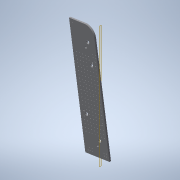
# Autodesk Inventor part: inside wall
Saved by Autodesk Inventor 2020 (Build 240168000, 168)
## iProperties
Created: 2019-10-13
Part Number: inside wall
Material: Generic
Document SubType Name: Modeling
Designer: ball
Density: 1 g/cm^3
Appearance: Default
Author: ball
Autodesk Inventor part; units mm, degrees
ref_plane "XZ Plane" through (0, 0, 0) normal (0, 1, 0) x (-1, 0, 0)
ref_plane "XY Plane" through (0, 0, 0) normal (0, 0, 1) x (1, 0, 0)
ref_plane "Work Plane1" through (-0.0003, 0.0023, 0) normal (0, 0, 1) x (1, 0, 0)
sketch "Sketch1" plane through (-0.0003, 0.0023, 0) normal (0, 0, 1) x (1, 0, 0)
  circle A0 centre (0.0003, -0.0023) radius 6.3373 construction
  circle A1 centre (-49.0975, 326.5271) radius 6.3373 construction
  circle A2 centre (0.0003, -0.0023) radius 6.4516
  circle A3 centre (-49.0975, 326.5271) radius 6.4516
  circle A4 centre (-49.0975, 326.5271) radius 60.325 construction
  circle A5 centre (0.0003, -0.0023) radius 60.325 construction
  circle A6 centre (0.0003, -0.0023) radius 31.75 construction
  circle A7 centre (-49.0975, 326.5271) radius 31.75 construction
  line L0 (-58.7973, -69.8464) -> (40.3672, -54.9357)
  line L1 (-125.8347, 375.9918) -> (-58.0673, 386.1815)
  circle A8 centre (-54.0299, 68.9302) radius 6.3373 construction
  circle A9 centre (-36.6118, 251.3479) radius 6.3373 construction
  circle A10 centre (-54.0299, 68.9302) radius 6.4516
  line L2 (-82.6344, 131.3852) -> (-87.6899, 165.0073) construction
  line L3 (-58.7973, -69.8464) -> (-125.8347, 375.9918)
  arc A11 (-21.1234, 354.0125) -> (-58.0673, 386.1815) centre (-58.7307, 348.1214) ccw
  line L4 (40.3672, -54.9357) -> (-21.1234, 354.0125)
  circle A12 centre (-32.9949, 251.8918) radius 6.3373 construction
  circle A13 centre (-32.9949, 251.8918) radius 6.4516
  point P0 (0.0003, -0.0023)
  dimension "d11" = 120.65
  dimension "d0" = 12.9032
  dimension "d3" = 12.9032
  dimension "d13" = 120.65
  dimension "d14" = 63.5
  dimension "d16" = 63.5
  dimension "d19" = 12.9032
  dimension "d81" = 12.9032
  constraints: 10 end point, 9 centre point, 8 coincident, 3 tangent, 2 point on circle, 9 other
  measures "d0" diameter of A2
  measures "d3" diameter of A3
  measures "d13" diameter of A5
  measures "d14" diameter of A6
  measures "d16" diameter of A7
  measures "d19" diameter of A10
  measures "d81" diameter of A13
extrude "Extrusion1" add sketch "Sketch1" along normal blind 6.35 contours L3 L1 A11 L4 L0 | A13
sketch "Sketch2" plane through (-0.0003, 0.0023, 6.35) normal (0, 0, 1) x (1, 0, 0)
  circle A0 centre (-59.5704, 139.9475) radius 1.9685 construction
  circle A1 centre (-64.857, 175.1068) radius 1.9685 construction
  circle A2 centre (-25.7636, 145.0307) radius 1.9685 construction
  circle A3 centre (-31.0502, 180.1901) radius 1.9685 construction
  circle A4 centre (-59.5704, 139.9475) radius 1.778
  circle A5 centre (-64.857, 175.1068) radius 1.778
  circle A6 centre (-25.7636, 145.0307) radius 1.778
  circle A7 centre (-31.0502, 180.1901) radius 1.778
  circle A8 centre (-48.1268, -55.3992) radius 1.778
  line L0 (-58.7973, -69.8464) -> (40.3672, -54.9357) projected
  line L1 (-125.8347, 375.9918) -> (-58.7973, -69.8464) projected
  circle A9 centre (-111.3879, 365.3242) radius 1.778
  line L2 (-58.0673, 386.1815) -> (-125.8347, 375.9918) projected
  circle A10 centre (-77.9428, 262.471) radius 1.778
  point P0 (0.0003, -0.0023)
  point P1 (-26.6702, 390.9025)
  dimension "d24" = 3.556
  dimension "d25" = 3.556
  dimension "d26" = 3.556
  dimension "d27" = 3.556
  dimension "d28" = 3.556
  dimension "d29" = 12.7
  dimension "d30" = 12.7
  dimension "d31" = 3.556
  dimension "d32" = 12.6972
  dimension "d33" = 12.7
  dimension "d34" = 3.556
  dimension "d35" = 30.48
  dimension "d36" = 119.38
  constraints: 7 centre point, 4 coincident
  measures "d24" diameter of A4
  measures "d25" diameter of A5
  measures "d26" diameter of A6
  measures "d27" diameter of A7
  measures "d28" diameter of A8
  measures "d29" distance from line of L0 A8.centre
  measures "d30" distance from line of L1 A8.centre
  measures "d31" diameter of A9
  measures "d32" distance from line of L2 A9.centre
  measures "d33" distance from line of L1 A9.centre
  measures "d34" diameter of A10
  measures "d35" distance from line of L1 A10.centre
  measures "d36" distance from line of L2 A10.centre
extrude "Extrusion2" cut sketch "Sketch2" against normal up to surface (6.35 mm away)
sketch "Sketch3" plane through (-0.0003, 0.0023, 6.35) normal (0, 0, 1) x (1, 0, 0)
  circle A0 centre (-32.2734, 257.2219) radius 3.048 construction
  circle A1 centre (-57.7822, 304.4219) radius 4.25 construction
  circle A2 centre (-59.904, 73.2686) radius 3.048 construction
  circle A3 centre (-8.6844, -22.1075) radius 4.25 construction
  circle A4 centre (-57.7822, 304.4219) radius 4.25
  circle A5 centre (-30.2618, 263.525) radius 3.175
  circle A6 centre (-65.0875, 76.3166) radius 3.048
  circle A7 centre (-8.6844, -22.1075) radius 4.25
  line L0 (40.3672, -54.9357) -> (-21.1234, 354.0125) projected
  line L1 (-58.0673, 386.1815) -> (-125.8347, 375.9918) projected
  arc A8 (-34.3449, 253.3797) -> (-33.8476, 250.0726) centre (-36.6118, 251.3479) ccw projected
  arc A9 (-56.2968, 66.8984) -> (-56.7941, 70.2055) centre (-54.0299, 68.9302) ccw projected
  point P0 (0.0003, -0.0023)
  point P1 (-26.6702, 390.9025)
  dimension "d41" = 12.1771
  dimension "d42" = 6.35
  dimension "d43" = 7.3865
  dimension "d44" = 11.0576
  constraints: 4 centre point, 2 coincident, 2 concentric
  measures "d41" vertical distance of A8.centre A5.centre
  measures "d42" horizontal distance of A8.centre A5.centre
  measures "d43" vertical distance of A6.centre A9.centre
  measures "d44" horizontal distance of A6.centre A9.centre
extrude "Extrusion3" cut sketch "Sketch3" against normal through all
sketch "Sketch4" plane through (-0.0003, 0.0023, 6.35) normal (0, 0, 1) x (1, 0, 0)
  arc A0 (-29.6539, 293.2296) -> (-29.0598, 294.034) centre (-28.4354, 292.9511) ccw construction
  arc A1 (-27.2269, 281.8437) -> (-28.0313, 282.4378) centre (-26.9484, 283.0623) ccw construction
  arc A2 (-15.841, 284.2708) -> (-16.4351, 283.4664) centre (-17.0596, 284.5492) ccw construction
  arc A3 (-18.2681, 295.6566) -> (-17.4637, 295.0625) centre (-18.5465, 294.4381) ccw construction
  circle A4 centre (-26.9484, 283.0623) radius 1.7
  circle A5 centre (-28.4354, 292.9511) radius 1.7
  circle A6 centre (-17.0596, 284.5492) radius 1.7
  circle A7 centre (-18.5465, 294.4381) radius 1.7
  circle A8 centre (-26.9484, 283.0623) radius 1.7
  circle A9 centre (-28.4354, 292.9511) radius 1.7
  circle A10 centre (-17.0596, 284.5492) radius 1.7
  circle A11 centre (-18.5465, 294.4381) radius 1.7
  circle A12 centre (-40.0242, -53.8744) radius 1.7
  circle A13 centre (-41.5111, -43.9856) radius 1.7
  circle A14 centre (-30.1354, -52.3875) radius 1.7
  circle A15 centre (-31.6223, -42.4987) radius 1.7
  circle A16 centre (18.6862, -43.9856) radius 1.7
  circle A17 centre (17.1993, -34.0967) radius 1.7
  circle A18 centre (28.575, -42.4987) radius 1.7
  circle A19 centre (27.0881, -32.6098) radius 1.7
  point P0 (0.0003, -0.0023)
  dimension "d47" = 3.4
  dimension "d48" = 3.4
  dimension "d49" = 3.4
  dimension "d50" = 3.4
  dimension "d51" = 3.4
  dimension "d52" = 3.4
  dimension "d53" = 3.4
  dimension "d54" = 3.4
  dimension "d55" = 3.4
  dimension "d56" = 3.4
  dimension "d57" = 3.4
  dimension "d58" = 3.4
  dimension "d59" = 3.4
  dimension "d60" = 3.4
  dimension "d61" = 3.4
  dimension "d62" = 3.4
  constraints: 16 centre point, 4 coincident
  measures "d47" diameter of A4
  measures "d48" diameter of A5
  measures "d49" diameter of A6
  measures "d50" diameter of A7
  measures "d51" diameter of A8
  measures "d52" diameter of A9
  measures "d53" diameter of A10
  measures "d54" diameter of A11
  measures "d55" diameter of A12
  measures "d56" diameter of A13
  measures "d57" diameter of A14
  measures "d58" diameter of A15
  measures "d59" diameter of A16
  measures "d60" diameter of A17
  measures "d61" diameter of A18
  measures "d62" diameter of A19
extrude "Extrusion4" cut sketch "Sketch4" against normal through all
sketch "Sketch5" plane through (-0.0003, 0.0023, 6.35) normal (0, 0, 1) x (1, 0, 0)
  circle A0 centre (9.1502, 60.0002) radius 2.25 construction
  circle A1 centre (9.1502, 60.0002) radius 2.1
  point P0 (0.0003, -0.0023)
  dimension "d65" = 4.2
  constraints: 2 centre point, 1 coincident, 2 other
  measures "d65" diameter of A1
extrude "Extrusion5" cut sketch "Sketch5" against normal through all
sketch "Sketch6" plane through (-0.0003, 0.0023, 6.35) normal (0, 0, 1) x (1, 0, 0)
  circle A0 centre (18.9899, 18.9065) radius 1.778
  line L0 (40.3672, -54.9357) -> (-21.1234, 354.0125) projected
  line L1 (-58.7973, -69.8464) -> (40.3672, -54.9357) projected
  circle A1 centre (17.1015, 31.4653) radius 1.778
  circle A2 centre (15.2131, 44.0241) radius 1.778
  circle A3 centre (13.3247, 56.583) radius 1.778
  circle A4 centre (11.4363, 69.1418) radius 1.778
  circle A5 centre (9.548, 81.7006) radius 1.778
  circle A6 centre (7.6596, 94.2594) radius 1.778
  circle A7 centre (5.7712, 106.8182) radius 1.778
  circle A8 centre (3.8828, 119.3771) radius 1.778
  circle A9 centre (1.9945, 131.9359) radius 1.778
  circle A10 centre (0.1061, 144.4947) radius 1.778
  circle A11 centre (-1.7823, 157.0535) radius 1.778
  circle A12 centre (-3.6707, 169.6124) radius 1.778
  circle A13 centre (-5.5591, 182.1712) radius 1.778
  circle A14 centre (-7.4474, 194.73) radius 1.778
  circle A15 centre (-9.3358, 207.2888) radius 1.778
  circle A16 centre (-11.2242, 219.8477) radius 1.778
  circle A17 centre (-13.1126, 232.4065) radius 1.778
  circle A18 centre (-15.0009, 244.9653) radius 1.778
  circle A19 centre (-16.8893, 257.5241) radius 1.778
  circle A20 centre (-18.7777, 270.0829) radius 1.778
  circle A21 centre (-20.6661, 282.6418) radius 1.778
  circle A22 centre (6.431, 17.0181) radius 1.778
  circle A23 centre (4.5427, 29.5769) radius 1.778
  circle A24 centre (2.6543, 42.1358) radius 1.778
  circle A25 centre (0.7659, 54.6946) radius 1.778
  circle A26 centre (-1.1225, 67.2534) radius 1.778
  circle A27 centre (-3.0109, 79.8122) radius 1.778
  circle A28 centre (-4.8992, 92.371) radius 1.778
  circle A29 centre (-6.7876, 104.9299) radius 1.778
  circle A30 centre (-8.676, 117.4887) radius 1.778
  circle A31 centre (-10.5644, 130.0475) radius 1.778
  circle A32 centre (-12.4527, 142.6063) radius 1.778
  circle A33 centre (-14.3411, 155.1652) radius 1.778
  circle A34 centre (-16.2295, 167.724) radius 1.778
  circle A35 centre (-18.1179, 180.2828) radius 1.778
  circle A36 centre (-20.0063, 192.8416) radius 1.778
  circle A37 centre (-21.8946, 205.4005) radius 1.778
  circle A38 centre (-23.783, 217.9593) radius 1.778
  circle A39 centre (-25.6714, 230.5181) radius 1.778
  circle A40 centre (-27.5598, 243.0769) radius 1.778
  circle A41 centre (-29.4481, 255.6357) radius 1.778
  circle A42 centre (-31.3365, 268.1946) radius 1.778
  circle A43 centre (-33.2249, 280.7534) radius 1.778
  circle A44 centre (-6.1278, 15.1297) radius 1.778
  circle A45 centre (-8.0162, 27.6886) radius 1.778
  circle A46 centre (-9.9045, 40.2474) radius 1.778
  circle A47 centre (-11.7929, 52.8062) radius 1.778
  circle A48 centre (-13.6813, 65.365) radius 1.778
  circle A49 centre (-15.5697, 77.9238) radius 1.778
  circle A50 centre (-17.4581, 90.4827) radius 1.778
  circle A51 centre (-19.3464, 103.0415) radius 1.778
  circle A52 centre (-21.2348, 115.6003) radius 1.778
  circle A53 centre (-23.1232, 128.1591) radius 1.778
  circle A54 centre (-25.0116, 140.718) radius 1.778
  circle A55 centre (-26.8999, 153.2768) radius 1.778
  circle A56 centre (-28.7883, 165.8356) radius 1.778
  circle A57 centre (-30.6767, 178.3944) radius 1.778
  circle A58 centre (-32.5651, 190.9533) radius 1.778
  circle A59 centre (-34.4535, 203.5121) radius 1.778
  circle A60 centre (-36.3418, 216.0709) radius 1.778
  circle A61 centre (-38.2302, 228.6297) radius 1.778
  circle A62 centre (-40.1186, 241.1885) radius 1.778
  circle A63 centre (-42.007, 253.7474) radius 1.778
  circle A64 centre (-43.8953, 266.3062) radius 1.778
  circle A65 centre (-45.7837, 278.865) radius 1.778
  circle A66 centre (-18.6866, 13.2414) radius 1.778
  circle A67 centre (-20.575, 25.8002) radius 1.778
  circle A68 centre (-22.4634, 38.359) radius 1.778
  circle A69 centre (-24.3517, 50.9178) radius 1.778
  circle A70 centre (-26.2401, 63.4766) radius 1.778
  circle A71 centre (-28.1285, 76.0355) radius 1.778
  circle A72 centre (-30.0169, 88.5943) radius 1.778
  circle A73 centre (-31.9053, 101.1531) radius 1.778
  circle A74 centre (-33.7936, 113.7119) radius 1.778
  circle A75 centre (-35.682, 126.2708) radius 1.778
  circle A76 centre (-37.5704, 138.8296) radius 1.778
  circle A77 centre (-39.4588, 151.3884) radius 1.778
  circle A78 centre (-41.3471, 163.9472) radius 1.778
  circle A79 centre (-43.2355, 176.5061) radius 1.778
  circle A80 centre (-45.1239, 189.0649) radius 1.778
  circle A81 centre (-47.0123, 201.6237) radius 1.778
  circle A82 centre (-48.9007, 214.1825) radius 1.778
  circle A83 centre (-50.789, 226.7413) radius 1.778
  circle A84 centre (-52.6774, 239.3002) radius 1.778
  circle A85 centre (-54.5658, 251.859) radius 1.778
  circle A86 centre (-56.4542, 264.4178) radius 1.778
  circle A87 centre (-58.3425, 276.9766) radius 1.778
  circle A88 centre (-31.2454, 11.353) radius 1.778
  circle A89 centre (-33.1338, 23.9118) radius 1.778
  circle A90 centre (-35.0222, 36.4706) radius 1.778
  circle A91 centre (-36.9106, 49.0294) radius 1.778
  circle A92 centre (-38.7989, 61.5883) radius 1.778
  circle A93 centre (-40.6873, 74.1471) radius 1.778
  circle A94 centre (-42.5757, 86.7059) radius 1.778
  circle A95 centre (-44.4641, 99.2647) radius 1.778
  circle A96 centre (-46.3525, 111.8236) radius 1.778
  circle A97 centre (-48.2408, 124.3824) radius 1.778
  circle A98 centre (-50.1292, 136.9412) radius 1.778
  circle A99 centre (-52.0176, 149.5) radius 1.778
  circle A100 centre (-53.906, 162.0589) radius 1.778
  circle A101 centre (-55.7943, 174.6177) radius 1.778
  circle A102 centre (-57.6827, 187.1765) radius 1.778
  circle A103 centre (-59.5711, 199.7353) radius 1.778
  circle A104 centre (-61.4595, 212.2941) radius 1.778
  circle A105 centre (-63.3479, 224.853) radius 1.778
  circle A106 centre (-65.2362, 237.4118) radius 1.778
  circle A107 centre (-67.1246, 249.9706) radius 1.778
  circle A108 centre (-69.013, 262.5294) radius 1.778
  circle A109 centre (-70.9014, 275.0883) radius 1.778
  circle A110 centre (-43.8043, 9.4646) radius 1.778
  circle A111 centre (-45.6926, 22.0234) radius 1.778
  circle A112 centre (-47.581, 34.5822) radius 1.778
  circle A113 centre (-49.4694, 47.1411) radius 1.778
  circle A114 centre (-51.3578, 59.6999) radius 1.778
  circle A115 centre (-53.2461, 72.2587) radius 1.778
  circle A116 centre (-55.1345, 84.8175) radius 1.778
  circle A117 centre (-57.0229, 97.3764) radius 1.778
  circle A118 centre (-58.9113, 109.9352) radius 1.778
  circle A119 centre (-60.7997, 122.494) radius 1.778
  circle A120 centre (-62.688, 135.0528) radius 1.778
  circle A121 centre (-64.5764, 147.6117) radius 1.778
  circle A122 centre (-66.4648, 160.1705) radius 1.778
  circle A123 centre (-68.3532, 172.7293) radius 1.778
  circle A124 centre (-70.2415, 185.2881) radius 1.778
  circle A125 centre (-72.1299, 197.8469) radius 1.778
  circle A126 centre (-74.0183, 210.4058) radius 1.778
  circle A127 centre (-75.9067, 222.9646) radius 1.778
  circle A128 centre (-77.7951, 235.5234) radius 1.778
  circle A129 centre (-79.6834, 248.0822) radius 1.778
  circle A130 centre (-81.5718, 260.6411) radius 1.778
  circle A131 centre (-83.4602, 273.1999) radius 1.778
  circle A132 centre (-56.3631, 7.5762) radius 1.778
  circle A133 centre (-58.2515, 20.135) radius 1.778
  circle A134 centre (-60.1398, 32.6939) radius 1.778
  circle A135 centre (-62.0282, 45.2527) radius 1.778
  circle A136 centre (-63.9166, 57.8115) radius 1.778
  circle A137 centre (-65.805, 70.3703) radius 1.778
  circle A138 centre (-67.6933, 82.9292) radius 1.778
  circle A139 centre (-69.5817, 95.488) radius 1.778
  circle A140 centre (-71.4701, 108.0468) radius 1.778
  circle A141 centre (-73.3585, 120.6056) radius 1.778
  circle A142 centre (-75.2469, 133.1644) radius 1.778
  circle A143 centre (-77.1352, 145.7233) radius 1.778
  circle A144 centre (-79.0236, 158.2821) radius 1.778
  circle A145 centre (-80.912, 170.8409) radius 1.778
  circle A146 centre (-82.8004, 183.3997) radius 1.778
  circle A147 centre (-84.6887, 195.9586) radius 1.778
  circle A148 centre (-86.5771, 208.5174) radius 1.778
  circle A149 centre (-88.4655, 221.0762) radius 1.778
  circle A150 centre (-90.3539, 233.635) radius 1.778
  circle A151 centre (-92.2423, 246.1939) radius 1.778
  circle A152 centre (-94.1306, 258.7527) radius 1.778
  circle A153 centre (-96.019, 271.3115) radius 1.778
  point P0 (0.0003, -0.0023)
  dimension "d68" = 3.556
  dimension "d69" = 10.16
  dimension "d70" = 76.2
  dimension "d73" = 12.7
  dimension "d76" = 12.7
  constraints: 154 centre point, 308 other
  measures "d68" diameter of A0
  measures "d69" distance from line of L0 A0.centre
  measures "d70" distance from line of L1 A0.centre
  measures "d73" distance of A0.centre A1.centre
  measures "d76" distance of A0.centre A22.centre
extrude "Extrusion6" cut sketch "Sketch6" against normal through all contours A0 | A1 | A2 | A4 | A5 | A6 | A7 | A8 | A9 | A10 | A11 | A12 | A13 | A14 | A15 | A16 | A17 | A18 | A19 | A20 | A22 | A23 | A24 | A25 | A26 | A27 | A28 | A29 | A30 | A31 | A32 | A33 | A34 | A35 | A36 | A37 | A38 | A39 | A40 | A44 | A45 | A46 | A47 | A48 | A49 | A50 | A51 | A52 | A53 | A55 | A56 | A58 | A59 | A60 | A61 | A64 | A65 | A66 | A67 | A68 | A69 | A70 | A71 | A72 | A73 | A74 | A75 | A76 | A77 | A78 | A79 | A80 | A81 | A82 | A83 | A84 | A85 | A86 | A87 | A88 | A89 | A90 | A91 | A92 | A93 | A94 | A95 | A96 | A97 | A98 | A99 | A100 | A101 | A102 | A103 | A104 | A105 | A106 | A107 | A108 | A109 | A110 | A111 | A112 | A113 | A116 | A117 | A118 | A119 | A121 | A122 | A124 | A125 | A126 | A127 | A128 | A129 | A131 | A132 | A133 | A134 | A135 | A136 | A139 | A140 | A141 | A142 | A143 | A144 | A145 | A146 | A147 | A148 | A149 | A150 | A151 | A152 | A153
sketch "Sketch7" plane through (-0.0003, 0.0023, 6.35) normal (0, 0, 1) x (1, 0, 0)
  circle A0 centre (-32.9949, 251.8918) radius 6.9215 construction
  circle A1 centre (-32.9949, 251.8918) radius 6.4516
  point P0 (0.0003, -0.0023)
  dimension "d82" = 12.9032
  constraints: 2 centre point, 1 coincident, 2 other
  measures "d82" diameter of A1
extrude "Extrusion7" cut sketch "Sketch7" against normal through all
sketch "Sketch8" plane through (-0.0003, 0.0023, 0) normal (0, 0, -1) x (-1, 0, 0)
  circle A0 centre (91.5803, 211.0567) radius 2 construction
  circle A1 centre (59.936, 215.8148) radius 2 construction
  circle A2 centre (77.306, 116.1239) radius 2 construction
  circle A3 centre (45.6617, 120.882) radius 2 construction
  circle A4 centre (91.5803, 211.0567) radius 1.778
  circle A5 centre (59.936, 215.8148) radius 1.778
  circle A6 centre (77.306, 116.1239) radius 1.778
  circle A7 centre (45.6617, 120.882) radius 1.778
  point P0 (-0.0003, -0.0023)
  dimension "d85" = 3.556
  dimension "d86" = 3.556
  dimension "d87" = 3.556
  dimension "d88" = 3.556
  constraints: 8 centre point, 4 coincident, 8 other
  measures "d85" diameter of A4
  measures "d86" diameter of A5
  measures "d87" diameter of A6
  measures "d88" diameter of A7
extrude "Extrusion8" cut sketch "Sketch8" against normal through all
sketch "Sketch9" plane through (-0.0003, 0.0023, 6.35) normal (0, 0, 1) x (1, 0, 0)
  arc A0 (-74.1387, 108.5102) -> (-78.0942, 107.9154) centre (-76.1164, 108.2128) ccw construction
  circle A1 centre (-76.1164, 108.2128) radius 3.175
  circle A2 centre (-44.4722, 112.9709) radius 2 construction
  circle A3 centre (-44.4722, 112.9709) radius 3.175
  point P0 (0.0003, -0.0023)
  dimension "d91" = 6.35
  dimension "d92" = 6.35
  constraints: 4 centre point, 2 coincident, 2 point on circle, 6 other
  measures "d91" diameter of A1
  measures "d92" diameter of A3
extrude "Extrusion9" cut sketch "Sketch9" against normal through all
equation "\"d0\" = d3"
equation "\"d19\" = d3"
body "Solid1"
